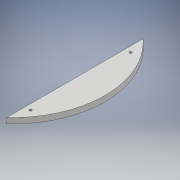
# Autodesk Inventor part: ガイド横v1
Saved by Autodesk Inventor 2018.3 (Build 223284000, 284)
## iProperties
Created: 2019-02-14
Part Number: ガイド横v1
Material: 一般
Document SubType Name: Modeling
Designer: shun2
Density: 1 g/cm^3
Appearance: 既定
Author: shun2
Autodesk Inventor part; units mm, degrees
ref_plane "YZ Plane" through (0, 0, 0) normal (1, 0, 0) x (0, 1, 0)
ref_plane "XZ Plane" through (0, 0, 0) normal (0, 1, 0) x (-1, 0, 0)
ref_plane "XY Plane" through (0, 0, 0) normal (0, 0, 1) x (1, 0, 0)
sketch "スケッチ1" plane through (0, 0, 0) normal (0, 0, 1) x (1, 0, 0)
  line L0 (0, 0) -> (0, 170)
  arc A0 (0, 0) -> (0, 170) centre (-77.4597, 85) ccw
  circle A1 centre (7, 22.5) radius 1.5
  circle A2 centre (7, 147.5) radius 1.5
  dimension "d0" = 170
  dimension "d1" = 115
  dimension "d2" = 3
  dimension "d3" = 3
  constraints: 3 centre point, 2 end point, 2 point on circle, 1 vertical
  measures "d0" distance of L0.start L0.end
  measures "d1" radius of A0
  measures "d2" diameter of A1
  measures "d3" diameter of A2
extrude "押し出し1" add sketch "スケッチ1" along normal blind 7
